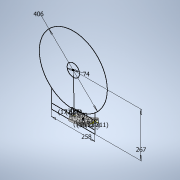
# Autodesk Inventor part: Layout
Saved by Autodesk Inventor 2022 (Build 260153070, 153G)
## iProperties
Created: 2021-11-12
Part Number: Layout
Material: Generic
Document SubType Name: Modeling
Designer: elmar
Density: 1 g/cm^3
Appearance: Default
Author: elmar
Autodesk Inventor part; units mm, degrees
ref_plane "YZ Plane" through (0, 0, 0) normal (1, 0, 0) x (0, 1, 0)
ref_plane "XZ Plane" through (0, 0, 0) normal (0, 1, 0) x (-1, 0, 0)
ref_plane "XY Plane" through (0, 0, 0) normal (0, 0, 1) x (1, 0, 0)
sketch "Sketch1" plane through (0, 0, 0) normal (0, 0, 1) x (1, 0, 0)
  circle A0 centre (0, 0) radius 203
  line L0 (-129, -156.7418) -> (-129, -267)
  line L1 (-129, -267) -> (129, -267)
  line L2 (129, -267) -> (129, -156.7418)
  circle A1 centre (0, 0) radius 37
  line L3 (0, -203) -> (0, -267)
  line L4 (0, -235) -> (-129, -235)
  line L5 (0, -235) -> (10.5, -235)
  dimension "d0" = 406
  dimension "d1" = 267
  dimension "d2" = 74
  dimension "d3" = 258
  dimension "d11" = 10.5
  dimension "HorizontalHalfAngle" = 2.558
  constraints: 12 end point, 3 perpendicular, 3 point on circle, 2 centre point, 2 coincident, 2 midpoint, 2 vertical, 1 horizontal, 1 parallel, 1 point on line
  measures "d0" diameter of A0
  measures "d1" distance from line of L1 point (0, 0)
  measures "d2" diameter of A1
  measures "d3" distance of L0.end L1.end
  measures "d11" distance of L4.start L5.end
extrude "Extrusion1" add sketch "Sketch1" along normal blind 74 contours A1
ref_plane "Work Plane1" through (0, -235, 0) normal (0, -1, 0) x (-1, 0, 0)
sketch "Sketch2" plane through (0, -235, 0) normal (0, -1, 0) x (-1, 0, 0)
  line L0 (0, 12.1244) -> (10.5, 6.0622)
  line L1 (10.5, 6.0622) -> (10.5, -6.0622)
  line L2 (10.5, -6.0622) -> (0, -12.1244)
  line L3 (0, -12.1244) -> (-10.5, -6.0622)
  line L4 (-10.5, -6.0622) -> (-10.5, 6.0622)
  line L5 (-10.5, 6.0622) -> (0, 12.1244)
  point P0 (0, 0)
  point P1 (0, 0)
  dimension "d8" = 21
  constraints: 12 end point, 1 coincident, 1 vertical, 13 other
  measures "d8" distance between parallel lines of L1 L4
extrude "Extrusion2" add sketch "Sketch2" along normal blind 2 draft 2.558 separate body
sketch "Sketch3" plane through (0, -235, 0) normal (0, 1, 0) x (1, 0, 0)
  line L0 (0, 0) -> (-5.2947, -9.1707)
  line L1 (-10.5894, -6.1138) -> (0, -12.2275) projected
  point P0 (-0.635, -1.0999)
  point P1 (-1.905, -3.2996)
  point P2 (-3.175, -5.4993)
  dimension "d16" = 1.27
  dimension "d17" = 2.54
  dimension "d18" = 2.54
  constraints: 3 point on line, 2 end point, 1 midpoint
  measures "d16" distance of L0.start point (-0.635, -1.1)
  measures "d17" distance of point (-0.635, -1.1) point (-1.905, -3.3)
  measures "d18" distance of point (-1.905, -3.3) point (-3.175, -5.499)
hole "Hole1" at (-1.905, -235, 3.2996) at (-0.635, -235, 1.0999) at (-3.175, -235, 5.4993) direction (0, -1, 0) diameter 0.7165 end through all bodies 2
pattern_circular "Circular Pattern1" count 7 over 30.7 about axis through (0, 0, -10) along (0, 0, 1) of "Extrusion2", "Hole1" bodies 2 skipped copies 4
ref_plane "Work Plane2" through (0, -235, -12.1244) normal (-0.0445035, 0.996031, 0.0770823) x (0.8660254, 0, 0.5)
sketch "Sketch4" plane through (0, -235, -12.1244) normal (-0.0445035, 0.996031, 0.0770823) x (0.8660254, 0, 0.5)
  line L0 (-0.0362, 20.979) -> (12.0761, 20.9999)
  line L1 (12.0761, 20.9999) -> (18.1503, 10.5208)
  line L2 (18.1503, 10.5208) -> (12.1123, 0.0209)
  line L3 (12.1123, 0.0209) -> (0, 0)
  line L4 (0, 0) -> (-6.0742, 10.4791)
  line L5 (-6.0742, 10.4791) -> (-0.0362, 20.979)
  point P0 (6.0622, 10.4583)
  point P1 (6.038, 10.5)
  constraints: 12 end point, 2 coincident, 13 other
extrude "Extrusion3" add sketch "Sketch4" against normal blind 2 draft 2.558 separate body
sketch "Sketch5" plane through (0, -235, -12.1244) normal (-0.0445035, 0.996031, 0.0770823) x (0.8660254, 0, 0.5)
  line L0 (6.0622, 10.4583) -> (6.0561, 0.0104)
  line L1 (0, 0) -> (12.1123, 0.0209) projected
  point P0 (6.0614, 9.1883)
  point P1 (6.06, 6.6483)
  point P2 (6.0585, 4.1083)
  dimension "d28" = 1.27
  dimension "d29" = 2.54
  dimension "d30" = 2.54
  constraints: 3 point on line, 2 end point, 1 midpoint
  measures "d28" distance of point (6.061, 9.188) L0.start
  measures "d29" distance of point (6.06, 6.648) point (6.061, 9.188)
  measures "d30" distance of point (6.059, 4.108) point (6.06, 6.648)
hole "Hole2" at (9.8253, -234.1822, -17.0194) at (8.5591, -234.4083, -14.8291) at (7.2928, -234.6343, -12.6389) direction (0.0445035, -0.996031, -0.0770823) diameter 0.7165 end through all bodies 3
pattern_circular "Circular Pattern2" count 6 over 25.583 about axis through (0, 0, -10) along (0, 0, 1) of "Extrusion3", "Hole2" bodies 3
mirror "Mirror1" about plane through (0, 0, 0) normal (0, 0, 1) of "Extrusion3", "Hole2", "Circular Pattern2" bodies 3
ref_plane "Work Plane3" through (111.0038, -207.5294, -30.4958) normal (0, 0, 1) x (-0.9643271, -0.2647136, 0)
sketch "Sketch6" plane through (111.0038, -207.5294, -30.4958) normal (0, 0, 1) x (-0.9643271, -0.2647136, 0)
  line L0 (0, 0) -> (10.1713, 2.7902) projected
  line L1 (10.1713, 2.7902) -> (20.6762, 3.7326) projected
  line L2 (10.1292, 2.7864) -> (10.1713, 2.7902) projected
  line L3 (20.6762, 3.7326) -> (31.0559, 5.6046) projected
  line L4 (31.0559, 5.6046) -> (41.6029, 5.6064) projected
  line L5 (41.6029, 5.6064) -> (52.1082, 6.5452) projected
  line L6 (52.1082, 6.5452) -> (62.6134, 5.6064) projected
  line L7 (62.6134, 5.6064) -> (73.1605, 5.6046) projected
  line L8 (73.1605, 5.6046) -> (83.5401, 3.7326) projected
  line L9 (83.5401, 3.7326) -> (94.045, 2.7902) projected
  line L10 (94.045, 2.7902) -> (104.2163, 0) projected
  line L11 (104.2163, 0) -> (114.6369, -1.8831) projected
  line L12 (-10.4206, -1.8831) -> (0, 0) projected
  arc A0 (117.2858, 7.7597) -> (-13.0694, 7.7597) centre (52.1082, -229.5104) ccw
  line L13 (-10.4206, -1.8831) -> (-13.0694, 7.7597)
  line L14 (-9.6711, -0.702) -> (-9.1417, -2.6306) projected
  line L15 (117.2858, 7.7597) -> (114.6369, -1.8831)
  dimension "d41" = 10
  constraints: 4 end point, 2 point on circle, 2 point on line, 1 centre point, 1 coincident
  measures "d41" distance of L12.start L13.end
extrude "Extrusion4" add sketch "Sketch6" along normal blind 10 separate body
fillet "Fillet1" radius 7 3 edges at (125.6611, -211.5526, -25.4958) (65.1353, -237.2817, -20.4958) (-0.0439, -246.0594, -25.4958)
mirror "Mirror2" about plane through (0, 0, 0) normal (0, 0, 1) of "Extrusion4", "Fillet1" bodies 4
ref_plane "Work Plane4" through (72.9487, -225.7424, 6.0622) normal (0.2647136, -0.9643271, 0) x (0, 0, 1)
ref_plane "Work Plane5" through (65.1353, -237.2817, 30.4958) normal (0.2647136, -0.9643271, 0) x (0.9643271, 0.2647136, 0)
sketch "Sketch7" plane through (65.1353, -237.2817, 30.4958) normal (0.2647136, -0.9643271, 0) x (0.9643271, 0.2647136, 0)
  line L0 (-10.5894, -24.382) -> (-10.5894, -36.6095) projected
  line L1 (10.5894, -36.6095) -> (10.5894, -24.382) projected
  line L2 (58.202, -57.9915) -> (-58.202, -57.9915) projected
  line L3 (58.202, -3) -> (-58.202, -3) projected
  line L4 (5, -3) -> (-5, -3)
  line L5 (-5, -3) -> (-5, -57.9915)
  line L6 (-5, -57.9915) -> (5, -57.9915)
  line L7 (5, -57.9915) -> (5, -3)
  line L8 (5, -3) -> (-5, -57.9915) construction
  line L9 (-5, -3) -> (5, -57.9915) construction
  line L10 (12.7, -21.6058) -> (-12.7, -21.6058)
  line L11 (-12.7, -21.6058) -> (-12.7, -39.3858)
  line L12 (-12.7, -39.3858) -> (12.7, -39.3858)
  line L13 (12.7, -39.3858) -> (12.7, -21.6058)
  line L14 (12.7, -21.6058) -> (-12.7, -39.3858) construction
  line L15 (-12.7, -21.6058) -> (12.7, -39.3858) construction
  circle A0 centre (0, -30.4958) radius 6.015
  line L16 (10.16, -24.1458) -> (-10.16, -24.1458)
  line L17 (-10.16, -24.1458) -> (-10.16, -36.8458)
  line L18 (-10.16, -36.8458) -> (10.16, -36.8458)
  line L19 (10.16, -36.8458) -> (10.16, -24.1458)
  line L20 (10.16, -24.1458) -> (-10.16, -36.8458) construction
  line L21 (-10.16, -24.1458) -> (10.16, -36.8458) construction
  line L22 (0, -81.8907) -> (0, 64.4034) projected
  point P0 (0, -24.1458)
  point P1 (-5, -21.6058)
  point P2 (-5, -39.3858)
  point P3 (5, -57.9915)
  point P4 (5, -39.3858)
  point P5 (5, -21.6058)
  point P6 (-5, -3)
  dimension "d45" = 10
  dimension "d46" = 12.03
  dimension "d47" = 25.4
  dimension "d48" = 17.78
  dimension "d49" = 12.7
  dimension "d50" = 20.32
  dimension "d51" = 2.54
  constraints: 36 end point, 6 midpoint, 6 parallel, 3 horizontal, 3 perpendicular, 2 point on line, 1 centre point, 1 coincident
  measures "d45" distance between parallel lines of L7 L5
  measures "d46" diameter of A0
  measures "d47" distance of L11.end L12.end
  measures "d48" distance of L10.end L11.end
  measures "d49" distance of L18.end L16.start
  measures "d50" distance of L16.start L16.end
  measures "d51" distance from line of point (0, -24.146) L10
extrude "Extrusion5" add sketch "Sketch7" against normal blind 2 contours L2 L22 L12 L7 | L2 L5 L12 L22 | L12 L22 L18 L7 | L7 L18 L19 L16 L10 L13 L12 | L12 L5 L18 L22 | L18 L22 A0 L7 | L7 A0 L16 L19 L18 | L12 L11 L10 L5 L16 L17 L18 | L18 L5 A0 L22 | L18 L17 L16 L5 A0 | A0 L22 L16 L7 | L10 L22 L3 L7 | L7 L16 L22 L10 | A0 L5 L16 L22 | L22 L16 L5 L10 | L10 L5 L3 L22 bodies 4
hole "Hole3" at (65.1353, -237.2817, 6.35) direction (-0.2647136, 0.9643271, 0) diameter 0.7165 depth 2 tip angle 118 bodies 4
pattern_linear "Rectangular Pattern1" count 5 spacing 2.54 along (-0.9643271, -0.2647136, 0) of "Hole3" first direction both ways yes bodies 4
hole "Hole4" at (55.3377, -239.9712, -6.35) at (55.3377, -239.9712, 6.35) at (74.9328, -234.5922, 6.35) at (74.9328, -234.5922, -6.35) direction (-0.2647136, 0.9643271, 0) diameter 2.5 depth 2 tip angle 118 bodies 4
sketch "Sketch8" plane through (0, 0, 0) normal (0, 0, 1) x (1, 0, 0)
  line L0 (-10.5894, -196.7049) -> (130.1035, -196.7049)
  line L1 (130.1035, -196.7049) -> (130.1035, -245.9581)
  line L2 (130.1035, -245.9581) -> (-10.5894, -245.9581)
  line L3 (-10.5894, -245.9581) -> (-10.5894, -196.7049)
  line L4 (-10.5894, -196.7049) -> (130.1035, -245.9581) construction
  line L5 (130.1035, -196.7049) -> (-10.5894, -245.9581) construction
  arc A0 (-0.0426, -238.9569) -> (7.1611, -245.9551) centre (6.9574, -238.9581) ccw projected
  arc A1 (119.4127, -215.1414) -> (122.0339, -205.4461) centre (116.0156, -209.021) ccw projected
  line L6 (-0.0421, -236.0594) -> (-0.0426, -238.9569) projected
  arc A2 (7.1611, -245.9551) -> (119.4127, -215.1414) centre (0, 0) ccw projected
  line L7 (122.0339, -205.4461) -> (120.5542, -202.9549) projected
  line L8 (62.7371, -228.5455) -> (62.2077, -226.6169) projected
  line L9 (62.7371, -228.5455) -> (64.6058, -235.3531)
  line L10 (64.2604, -235.4479) -> (64.9513, -235.2582) projected
  point P0 (0, 0)
  point P1 (59.7571, -221.3315)
  point P2 (-10.5894, -237)
  point P3 (130.1035, -198.379)
  point P4 (129.0056, -196.7049)
  point P5 (64.725, -235.3203)
  point P6 (64.4867, -235.3858)
  point P7 (63.6715, -231.9493)
  dimension "d71" = 56.2585
  dimension "d72" = 52.7997
  dimension "d73" = 17.6266
  dimension "d74" = 12.3105
  dimension "d75" = 3.9144
  dimension "d76" = 10.6178
  constraints: 14 end point, 4 midpoint, 3 point on line, 2 parallel, 1 horizontal, 1 perpendicular, 1 tangent
  measures "d71" horizontal distance of A1.centre point (59.757, -221.331)
  measures "d72" horizontal distance of A0.centre point (59.757, -221.331)
  measures "d73" vertical distance of A0.centre point (59.757, -221.331)
  measures "d74" vertical distance of A1.centre point (59.757, -221.331)
  measures "d75" horizontal distance of point (59.757, -221.331) point (63.671, -231.949)
  measures "d76" vertical distance of point (59.757, -221.331) point (63.671, -231.949)
equation "\"d10\" = HorizontalHalfAngle"
equation "\"d14\" = 12 * HorizontalHalfAngle"
equation "\"d27\" = HorizontalHalfAngle"
equation "\"d39\" = 10 * HorizontalHalfAngle"
body "Solid1"
body "Solid2"
body "Solid3"
body "Solid4"
